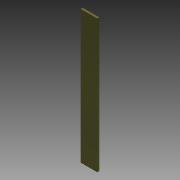
# Autodesk Inventor part: Part1
Saved by Autodesk Inventor 2013 (Build 170138000, 138)
## iProperties
Created: 2013-02-18
Part Number: Part1
Material: Titanium
Document SubType Name: Modeling
Designer: Arpan
Mass: 591.245 g
Surface Area: 470.967 cm^2
Volume: 131.097 cm^3
Density: 4.51 g/cm^3
Author: Arpan
Autodesk Inventor part; units mm, degrees
ref_plane "YZ Plane" through (0, 0, 0) normal (1, 0, 0) x (0, 1, 0)
ref_plane "XZ Plane" through (0, 0, 0) normal (0, 1, 0) x (-1, 0, 0)
ref_plane "XY Plane" through (0, 0, 0) normal (0, 0, 1) x (1, 0, 0)
sketch "Sketch1" plane through (0, 0, 0) normal (0, 0, 1) x (1, 0, 0)
  line L0 (0, 0) -> (0, 406.4)
  line L1 (0, 406.4) -> (-50.8, 406.4)
  line L2 (-50.8, 406.4) -> (-50.8, 0)
  line L3 (-50.8, 0) -> (0, 0)
  dimension "d0" = 406.4
  dimension "d1" = 50.8
  constraints: 8 end point, 2 perpendicular, 1 parallel, 1 vertical
  measures "d0" distance of L0.start L0.end
  measures "d1" distance of L0.end L1.end
extrude "Extrusion1" add sketch "Sketch1" along normal blind 6.35
body "Solid1"
